spool_cradle_bracket (Autodesk Fusion 360 design; units mm, degrees)
part number: 2026-09-02-15-56-20-841
Autodesk Fusion 360 part; units mm, degrees
sketch "Arm triangle" plane through (0, 0, 0) normal (0, 1, 0) x (1, 0, 0)
  line L0 (0, 0) -> (0, -90)
  line L1 (0, -90) -> (150, -90)
  line L2 (150, -90) -> (0, 0)
  dimension "d186" = 90
  constraint coincident L0.start L2.end
  constraint vertical L0
  constraint horizontal L1
  measures "d186" vertical distance of L0.start L0.end
extrude "Arm triangle (1)" add sketch "Arm triangle" along normal mid plane 24
sketch "Plate" plane through (0, 0, 0) normal (0, 1, 0) x (1, 0, 0)
  line L0 (0, 0) -> (6, 0)
  line L1 (6, 0) -> (6, -90)
  line L2 (6, -90) -> (0, -90)
  line L3 (0, -90) -> (0, 0)
  dimension "d190" = 6
  dimension "d191" = 90
  constraint coincident L0.start L3.end
  constraint horizontal L0
  constraint horizontal L2
  constraint vertical L1
  constraint vertical L3
  measures "d190" horizontal distance of L0.start L1.end
  measures "d191" vertical distance of L0.start L1.end
extrude "Plate (1)" add sketch "Plate" along normal mid plane 24
sketch "Lightening cutout" plane through (0, 0, 0) normal (0, 1, 0) x (1, 0, 0)
  line L0 (14, -24.7267) -> (14, -76)
  line L1 (14, -76) -> (37.3, -76)
  line L2 (37.3, -76) -> (37.3, -38.7067)
  line L3 (37.3, -38.7067) -> (14, -24.7267)
  dimension "d194" = 14
  dimension "d195" = 24.7267
  dimension "d196" = 76
  dimension "d197" = 37.3
  dimension "d198" = 38.7067
  constraint vertical L0
  constraint horizontal L1
  constraint vertical L2
  measures "d194" horizontal distance of origin L0.start
  measures "d195" vertical distance of origin L0.start
  measures "d196" vertical distance of origin L0.end
  measures "d197" horizontal distance of origin L1.end
  measures "d198" vertical distance of origin L2.end
extrude "Lightening cutout (1)" cut sketch "Lightening cutout" along normal mid plane 34
sketch "Saddle boss x=70" plane through (0, 0, 0) normal (0, 1, 0) x (1, 0, 0)
  circle A0 centre (70, -90) radius 22.7
  dimension "d201" = 70
  dimension "d202" = 90
  dimension "d203" = 45.4
  measures "d201" horizontal distance of origin A0.centre
  measures "d202" vertical distance of origin A0.centre
  measures "d203" diameter of A0
extrude "Saddle boss x=70 (1)" add sketch "Saddle boss x=70" along normal mid plane 24
sketch "Saddle boss x=150" plane through (0, 0, 0) normal (0, 1, 0) x (1, 0, 0)
  circle A0 centre (150, -90) radius 22.7
  dimension "d207" = 90
  dimension "d208" = 45.4
  measures "d207" vertical distance of origin A0.centre
  measures "d208" diameter of A0
extrude "Saddle boss x=150 (1)" add sketch "Saddle boss x=150" along normal mid plane 24
sketch "Rod pocket x=70" plane through (0, 0, 0) normal (0, 1, 0) x (1, 0, 0)
  circle A0 centre (70, -90) radius 17.1
  dimension "d211" = 70
  dimension "d212" = 90
  dimension "d213" = 34.2
  measures "d211" horizontal distance of origin A0.centre
  measures "d212" vertical distance of origin A0.centre
  measures "d213" diameter of A0
extrude "Rod pocket x=70 (1)" cut sketch "Rod pocket x=70" along normal mid plane 34
sketch "Drop-in opening x=70" plane through (0, 0, 0) normal (0, 1, 0) x (1, 0, 0)
  line L0 (52.9, -90) -> (87.1, -90)
  line L1 (87.1, -90) -> (87.1, -117.7)
  line L2 (87.1, -117.7) -> (52.9, -117.7)
  line L3 (52.9, -117.7) -> (52.9, -90)
  dimension "d216" = 52.9
  dimension "d217" = 90
  dimension "d218" = 87.1
  dimension "d219" = 117.7
  constraint horizontal L0
  constraint horizontal L2
  constraint vertical L1
  constraint vertical L3
  measures "d216" horizontal distance of origin L0.start
  measures "d217" vertical distance of origin L0.start
  measures "d218" horizontal distance of origin L1.end
  measures "d219" vertical distance of origin L1.end
extrude "Drop-in opening x=70 (1)" cut sketch "Drop-in opening x=70" along normal mid plane 34
sketch "Rod pocket x=150" plane through (0, 0, 0) normal (0, 1, 0) x (1, 0, 0)
  circle A0 centre (150, -90) radius 17.1
  dimension "d223" = 90
  dimension "d224" = 34.2
  measures "d223" vertical distance of origin A0.centre
  measures "d224" diameter of A0
extrude "Rod pocket x=150 (1)" cut sketch "Rod pocket x=150" along normal mid plane 34
sketch "Drop-in opening x=150" plane through (0, 0, 0) normal (0, 1, 0) x (1, 0, 0)
  line L0 (132.9, -90) -> (167.1, -90)
  line L1 (167.1, -90) -> (167.1, -117.7)
  line L2 (167.1, -117.7) -> (132.9, -117.7)
  line L3 (132.9, -117.7) -> (132.9, -90)
  dimension "d227" = 132.9
  dimension "d228" = 90
  dimension "d229" = 167.1
  dimension "d230" = 117.7
  constraint horizontal L0
  constraint horizontal L2
  constraint vertical L1
  constraint vertical L3
  measures "d227" horizontal distance of origin L0.start
  measures "d228" vertical distance of origin L0.start
  measures "d229" horizontal distance of origin L1.end
  measures "d230" vertical distance of origin L1.end
extrude "Drop-in opening x=150 (1)" cut sketch "Drop-in opening x=150" along normal mid plane 34
sketch "Hook profile" plane through (0, 0, 0) normal (0, 1, 0) x (1, 0, 0)
  line L0 (0, -88) -> (-8.3, -88)
  line L1 (-8.3, -88) -> (-8.3, -71)
  line L2 (-8.3, -71) -> (-5.3, -71)
  line L3 (-5.3, -71) -> (-3.8, -72.5)
  line L4 (-3.8, -72.5) -> (-3.8, -83)
  line L5 (-3.8, -83) -> (0, -83)
  line L6 (0, -83) -> (0, -88)
  dimension "d233" = 88
  dimension "d234" = 8.3
  dimension "d235" = 3.8
  dimension "d236" = 5
  dimension "d237" = 10.5
  dimension "d238" = 1.5
  dimension "d239" = 1.5
  constraint horizontal L0
  constraint horizontal L2
  constraint horizontal L5
  constraint vertical L1
  constraint vertical L4
  constraint vertical L6
  constraint coincident origin L6
  measures "d233" vertical distance of origin L0.start
  measures "d234" horizontal distance of L0.start L0.end
  measures "d235" horizontal distance of L4.end L5.end
  measures "d236" vertical distance of L0.start L5.end
  measures "d237" vertical distance of L3.end L4.end
  measures "d238" horizontal distance of L2.end L3.end
  measures "d239" vertical distance of L2.end L3.end
extrude "Hook profile (1)" add sketch "Hook profile" along normal mid plane 2.4
pattern_linear "Hook rows" count 4 spacing 25.4 along (0, 0, -1) count 3 spacing 0 along (0, 0, 1) of "Hook profile (1)"
equation "bracketWidth = 24.0 mm" comment "bracket width along the rods"
equation "hookTabWidth = slotWidth - 0.8 mm" comment "blade width through the slot"
equation "slotPitchVertical = 25.4 mm" comment "1 inch, measured"
equation "slotWidth = 3.2 mm" comment "measured slot width in the upright"
equation "faceMetalThickness = 2.0 mm" comment "upright face metal"
equation "hookThroat = faceMetalThickness + 1.8 mm" comment "gap behind the plate"
equation "hookNeckHeight = 5.0 mm" comment "bears on the slot bottom edge"
equation "hookLipThickness = 4.5 mm" comment "lip thickness behind the face"
equation "hookLipDrop = 12.0 mm" comment "engagement below the neck"
equation "plateThickness = 6.0 mm" comment "hook plate thickness"
equation "plateHeight = 90.0 mm" comment "plate height, also the rod height"
equation "rodOuterDiameter = 33.4 mm" comment "1 inch sch 40 PVC"
equation "saddleClearance = 0.8 mm" comment "diametral pocket clearance"
equation "saddleWall = 6.0 mm" comment "wall around the rod pocket"
equation "rearRodStandoff = 70.0 mm" comment "rear rod, from the upright"
equation "rodSpacing = 80.0 mm" comment "rod centres, front minus rear"
equation "memberWidth = 14.0 mm" comment "border around the lightening cutout"
equation "hookLipChamfer = 1.5 mm" comment "lead-in past slot burrs"
equation "topHookNeckTop = 88.0 mm" comment "top row, below the plate top"
equation "hookRows = 4" comment "number of hook rows (pattern count)"
equation "d186 = plateHeight"
equation "d187 = ( rearRodStandoff + rodSpacing )"
equation "d188 = bracketWidth"
equation "d190 = plateThickness"
equation "d191 = plateHeight"
equation "d192 = bracketWidth"
equation "d194 = memberWidth"
equation "d195 = plateHeight / ( rearRodStandoff + rodSpacing ) * ( ( memberWidth ) - ( -memberWidth * plateHeight / sqrt(( rearRodStandoff + rodSpacing ) * ( rearRodStandoff + rodSpacing ) + plateHeight * plateHeight) ) ) + ( memberWidth * ( rearRodStandoff + rodSpacing ) / sqrt(( rearRodStandoff + rodSpacing ) * ( rearRodStandoff + rodSpacing ) + plateHeight * plateHeight) )"
equation "d196 = plateHeight - memberWidth"
equation "d197 = rearRodStandoff - ( rodOuterDiameter + 2 * saddleWall ) / 2 - 10 mm"
equation "d198 = plateHeight / ( rearRodStandoff + rodSpacing ) * ( ( rearRodStandoff - ( rodOuterDiameter + 2 * saddleWall ) / 2 - 10 mm ) - ( -memberWidth * plateHeight / sqrt(( rearRodStandoff + rodSpacing ) * ( rearRodStandoff + rodSpacing ) + plateHeight * plateHeight) ) ) + ( memberWidth * ( rearRodStandoff + rodSpacing ) / sqrt(( rearRodStandoff + rodSpacing ) * ( rearRodStandoff + rodSpacing ) + plateHeight * plateHeight) )"
equation "d199 = bracketWidth + 10 mm"
equation "d201 = rearRodStandoff"
equation "d202 = plateHeight"
equation "d203 = rodOuterDiameter + 2 * saddleWall"
equation "d204 = bracketWidth"
equation "d206 = ( rearRodStandoff + rodSpacing )"
equation "d207 = plateHeight"
equation "d208 = rodOuterDiameter + 2 * saddleWall"
equation "d209 = bracketWidth"
equation "d211 = rearRodStandoff"
equation "d212 = plateHeight"
equation "d213 = rodOuterDiameter + saddleClearance"
equation "d214 = bracketWidth + 10 mm"
equation "d216 = rearRodStandoff - ( rodOuterDiameter + saddleClearance ) / 2"
equation "d217 = plateHeight"
equation "d218 = rearRodStandoff + ( rodOuterDiameter + saddleClearance ) / 2"
equation "d219 = plateHeight + ( rodOuterDiameter + 2 * saddleWall ) / 2 + 5 mm"
equation "d220 = bracketWidth + 10 mm"
equation "d222 = ( rearRodStandoff + rodSpacing )"
equation "d223 = plateHeight"
equation "d224 = rodOuterDiameter + saddleClearance"
equation "d225 = bracketWidth + 10 mm"
equation "d227 = ( rearRodStandoff + rodSpacing ) - ( rodOuterDiameter + saddleClearance ) / 2"
equation "d228 = plateHeight"
equation "d229 = ( rearRodStandoff + rodSpacing ) + ( rodOuterDiameter + saddleClearance ) / 2"
equation "d230 = plateHeight + ( rodOuterDiameter + 2 * saddleWall ) / 2 + 5 mm"
equation "d231 = bracketWidth + 10 mm"
equation "d233 = topHookNeckTop"
equation "d234 = hookThroat + hookLipThickness"
equation "d235 = hookThroat"
equation "d236 = hookNeckHeight"
equation "d237 = hookLipDrop - hookLipChamfer"
equation "d238 = hookLipChamfer"
equation "d239 = hookLipChamfer"
equation "d240 = hookTabWidth"
equation "d242 = hookRows"
equation "d244 = -slotPitchVertical"
named bodies: "spool_cradle_bracket"
